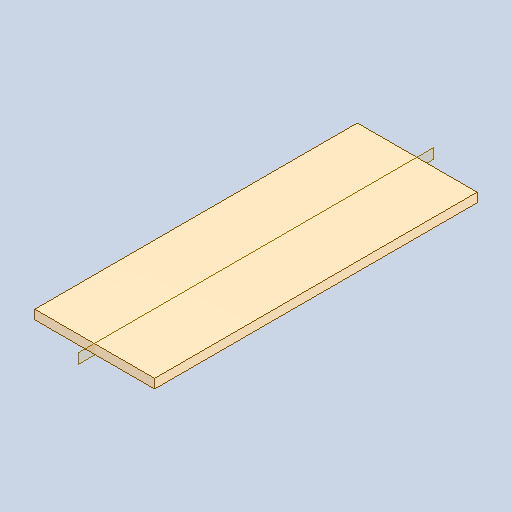
# Autodesk Inventor part: PCB
Saved by Autodesk Inventor 2026.2 (Build 302298010, 298A)
## iProperties
Created: 2026-04-26
Part Number: PCB
Material: Polyethylene, High Density
Document SubType Name: Modeling
Designer: piete
Density: 0.952 g/cm^3
Appearance: Smooth - Off-White
Author: piete
Autodesk Inventor part; units mm, degrees
ref_plane "XZ Plane" through (0, 0, 0) normal (0, 1, 0) x (-1, 0, 0)
ref_plane "XY Plane" through (0, 0, 0) normal (0, 0, 1) x (1, 0, 0)
sketch "Sketch1" plane through (0, 0, 0) normal (0, 1, 0) x (-1, 0, 0)
  line L0 (3.25, 8.75) -> (-3.25, 8.75)
  line L1 (-3.25, 8.75) -> (-3.25, -8.75)
  line L2 (-3.25, -8.75) -> (3.25, -8.75)
  line L3 (3.25, -8.75) -> (3.25, 8.75)
  point P0 (0, 0)
  dimension "d0" = 6.5
  dimension "d1" = 17.5
  dimension "d2" = 3.25
  dimension "d3" = 8.75
  constraints: 8 end point, 2 parallel, 1 horizontal, 1 perpendicular
  measures "d0" distance of L2.end L1.end
  measures "d1" distance of L1.end L0.end
  measures "d2" distance from line of point (0, 0) L3
  measures "d3" distance from line of L2 point (0, 0)
extrude "Extrusion1" add sketch "Sketch1" along normal blind 0.5
equation "\"d2\" = 0.5 * d0"
equation "\"d3\" = 0.5 * d1"
body "Solid1"
